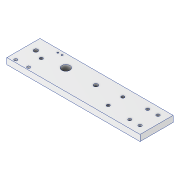
# Autodesk Inventor part: Columna Izquierda
Saved by Autodesk Inventor 2020 (Build 240168000, 168)
## iProperties
Created: 2020-05-17
Part Number: Columna Izquierda
Material: Aluminum 6061
Document SubType Name: Modeling
Designer: Pipi
Density: 2.7 g/cm^3
Appearance: Aluminum - Flat
Mass: 192.235 g
Surface Area: 470.037 cm^2
Volume: 192.235 cm^3
Author: Pipi
Autodesk Inventor part; units mm, degrees
ref_plane "YZ Plane" through (0, 0, 0) normal (1, 0, 0) x (0, 1, 0)
ref_plane "XZ Plane" through (0, 0, 0) normal (0, 1, 0) x (-1, 0, 0)
ref_plane "XY Plane" through (0, 0, 0) normal (0, 0, 1) x (1, 0, 0)
sketch "Boceto1" plane through (0, 0, 0) normal (0, 1, 0) x (-1, 0, 0)
  line L0 (6.1283, -21.2541) -> (6.1283, -85.7541)
  line L1 (6.1283, -85.7541) -> (-253.3717, -85.7541)
  line L2 (6.1283, -21.2541) -> (-253.3717, -21.2541)
  line L3 (-253.3717, -21.2541) -> (-253.3717, -85.7541)
  circle A0 centre (-127.3717, -61.2541) radius 4
  circle A1 centre (-10.3717, -61.2541) radius 4
  circle A2 centre (-68.8717, -61.2541) radius 8
  circle A3 centre (-35.3717, -79.2541) radius 1.5
  circle A4 centre (-43.3717, -79.2541) radius 1.5
  circle A5 centre (-28.8717, -53.2541) radius 3
  circle A6 centre (-173.3717, -67.7541) radius 3
  circle A7 centre (-173.3717, -39.2541) radius 3
  dimension "d0" = 64.5
  dimension "d22" = 8
  dimension "d23" = 8
  dimension "d27" = 16
  dimension "d103" = 58.5
  dimension "d104" = 117
  dimension "d105" = 3
  dimension "d106" = 3
  dimension "d115" = 6.5
  dimension "d121" = 259.5
  dimension "d122" = 126
  dimension "d128" = 6
  dimension "d129" = 35
  dimension "d130" = 32
  dimension "d131" = 6
  dimension "d132" = 6
  dimension "d133" = 80
  dimension "d134" = 18
  dimension "d135" = 80
  dimension "d136" = 18
  dimension "d143" = 40
  dimension "d144" = 40
  dimension "d145" = 40
  dimension "d149" = 8
  dimension "d150" = 41.5
  constraints: 8 centre point, 8 end point, 2 perpendicular, 1 horizontal, 1 vertical
  measures "d0" distance of L0.start L0.end
  measures "d22" diameter of A0
  measures "d23" diameter of A1
  measures "d27" diameter of A2
  measures "d103" distance of A2.centre A0.centre
  measures "d104" distance of A1.centre A0.centre
  measures "d105" diameter of A3
  measures "d106" diameter of A4
  measures "d115" distance from line of L1 A3.centre
  measures "d121" distance of L0.end L1.end
  measures "d122" distance from line of A0.centre L3
  measures "d128" diameter of A5
  measures "d129" distance from line of L0 A5.centre
  measures "d130" distance from line of L2 A5.centre
  measures "d131" diameter of A6
  measures "d132" diameter of A7
  measures "d133" distance from line of L3 A6.centre
  measures "d134" distance from line of L1 A6.centre
  measures "d135" distance from line of L3 A7.centre
  measures "d136" distance from line of L2 A7.centre
  measures "d143" distance from line of L2 A0.centre
  measures "d144" distance from line of L2 A2.centre
  measures "d145" distance from line of L2 A1.centre
  measures "d149" distance of A4.centre A3.centre
  measures "d150" distance from line of L0 A3.centre
extrude "Extrusion3" add sketch "Boceto1" along normal blind 12
sketch "Sketch2" plane through (0, 12, 0) normal (0, 1, 0) x (1, 0, 0)
  circle A0 centre (6.3717, 26.2541) radius 3
  line L0 (-6.1283, 21.2541) -> (253.3717, 21.2541) projected
  line L1 (-6.1283, 85.7541) -> (-6.1283, 21.2541) projected
  circle A1 centre (31.3717, 26.2541) radius 3
  circle A2 centre (218.3717, 71.2541) radius 3
  circle A3 centre (238.3717, 71.2541) radius 3
  circle A4 centre (218.3717, 36.2541) radius 3
  circle A5 centre (238.3717, 36.2541) radius 3
  line L2 (253.3717, 21.2541) -> (253.3717, 85.7541) projected
  line L3 (253.3717, 85.7541) -> (-6.1283, 85.7541) projected
  point P0 (253.3717, 20.7541)
  point P1 (-7.6283, 85.7541)
  dimension "d84" = 6
  dimension "d85" = 5
  dimension "d86" = 12.5
  dimension "d87" = 6
  dimension "d88" = 25
  dimension "d91" = 6
  dimension "d92" = 6
  dimension "d93" = 6
  dimension "d94" = 6
  dimension "d95" = 15
  dimension "d98" = 15
  dimension "d99" = 15
  dimension "d100" = 20
  dimension "d101" = 20
  dimension "d146" = 35
  dimension "d147" = 35
  dimension "d148" = 15
  constraints: 6 centre point, 2 other
  measures "d84" diameter of A0
  measures "d87" diameter of A1
  measures "d88" distance of A1.centre A0.centre
  measures "d91" diameter of A2
  measures "d92" diameter of A3
  measures "d93" diameter of A4
  measures "d94" diameter of A5
  measures "d95" distance from line of L2 A3.centre
  measures "d98" distance from line of L2 A5.centre
  measures "d100" distance of A4.centre A5.centre
  measures "d101" distance of A2.centre A3.centre
  measures "d146" distance of A4.centre A2.centre
  measures "d147" distance of A5.centre A3.centre
extrude "Extrusion4" cut sketch "Sketch2" against normal blind 25 contours A0 | A1 | A2 | A3 | A4 | A5
thread "Thread1" size "M3x0.5" class "6H" standard "ANSI Metric M Profile" length 40
thread "Thread2" size "M3x0.5" class "6H" standard "ANSI Metric M Profile" length 40
thread "Rosca3" size "M6x1" class "6H" standard "ISO Metric profile" length 922
thread "Rosca4" size "M6x1" class "6H" standard "ISO Metric profile" length 922
thread "Rosca5" size "M6x1" class "6H" standard "ISO Metric profile" length 922
body "Solid3"
